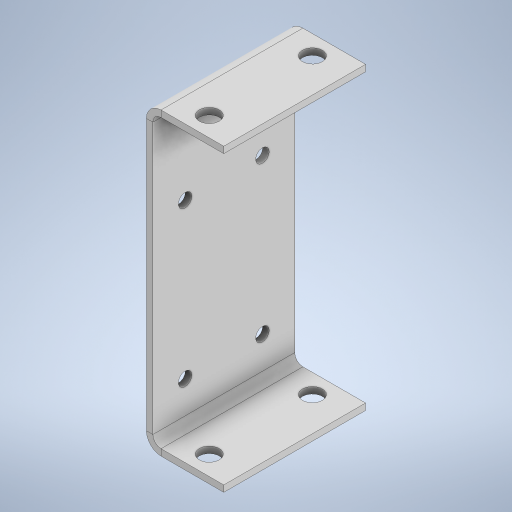
# Autodesk Inventor part: MotorSoport
Saved by Autodesk Inventor 2023.1 (Build 271208000, 208)
## iProperties
Created: 2022-09-08
Part Number: MotorSoport
Material: Genérico
Document SubType Name: Sheet Metal
Designer: Lab. de Manufactura
Density: 1 g/cm^3
Sheet Metal Rule: Por defecto_mm
Appearance: Valor por defecto
Flat Pattern Width: 2.2 cm
Flat Pattern Length: 6.67921 cm
Flat Pattern Area: 14.6943 cm^2
Sheet Metal Width: 22,000 mm
Sheet Metal Length: 66,792 mm
Sheet Metal Area: 1469,427 mm^2
Author: Lab. de Manufactura
Autodesk Inventor part; units mm, degrees
ref_plane "YZ Plane" through (0, 0, 0) normal (1, 0, 0) x (0, 1, 0)
ref_plane "XZ Plane" through (0, 0, 0) normal (0, 1, 0) x (-1, 0, 0)
ref_plane "XY Plane" through (0, 0, 0) normal (0, 0, 1) x (1, 0, 0)
sketch "Boceto1" plane through (0, 0, 0) normal (1, 0, 0) x (0, 1, 0)
  line L0 (0, 0) -> (46.5, 0)
  line L1 (46.5, 0) -> (46.5, -22)
  line L2 (46.5, -22) -> (0, -22)
  line L3 (0, -22) -> (0, 0)
  dimension "d0" = 46.5
  dimension "d1" = 22
  measures "d0" distance of L1.end L2.end
  measures "d1" distance of L0.end L1.end
extrude "Placa1" add sketch "Boceto1" along normal blind 1
sketch "Boceto2" plane through (0, 45.5, 0) normal (0, 1, 0) x (-1, 0, 0)
  line L0 (0, -22) -> (0, 0)
  line L1 (0, 0) -> (-12, 0)
  line L2 (-12, 0) -> (-12, -22)
  line L3 (-12, -22) -> (0, -22)
  constraints: 6 end point, 1 horizontal, 1 perpendicular, 1 vertical
edge flange "Pestaña1" height 12 angle 90 thickness 1 bend radius 1.27 thickness toward (0, 1, 0) relief tear relief width 1 relief depth 0.5 corner gap 1 corner form 0 edges at (1, 46.5, -11) (1, 0, -11) wall of the first edge with corners at (0, 45.5, -22) (0, 45.5, 0) (12, 45.5, 0) (12, 45.5, -22)
bend "Doblez1"
corner "Esquina1"
sketch "Boceto3" plane through (1, 0, 0) normal (1, 0, 0) x (0, 0, -1)
  circle A0 centre (17, 7.25) radius 1.05
  line L0 (0, 0) -> (22, 0) projected
  line L1 (0, 2.27) -> (0, 44.23) projected
  line L2 (0, 0) -> (22, 0) construction
  line L3 (11, 0) -> (11, 46.5) construction
  line L4 (22, 46.5) -> (0, 46.5) construction
  circle A1 centre (5, 7.25) radius 1.05
  line L5 (22, 44.23) -> (22, 2.27) projected
  circle A2 centre (17, 31.25) radius 1.05
  circle A3 centre (5, 31.25) radius 1.05
  dimension "d13" = 2.1
  dimension "d14" = 7.25
  dimension "d16" = 2.1
  dimension "d20" = 24
  dimension "d27" = 12
  dimension "d28" = 6
  constraints: 4 centre point, 2 end point, 2 midpoint, 1 horizontal alignment, 1 vertical, 4 other
  measures "d13" diameter of A0
  measures "d14" distance from line of L0 A0.centre
  measures "d16" diameter of A1
  measures "d20" distance of A0.centre A2.centre
  measures "d27" distance of A0.centre A1.centre
  measures "d28" distance from line of L3 A1.centre
extrude "Cortar1" cut sketch "Boceto3" against normal blind 1
sketch "Boceto4" plane through (12, 1, 0) normal (0, 1, 0) x (1, 0, 0)
  circle A0 centre (-5.25, 19) radius 1.55
  line L0 (-9.73, 22) -> (0, 22) projected
  line L1 (0, 0) -> (0, 22) construction
  line L2 (0, 11) -> (-13.2221, 11) construction
  circle A1 centre (-5.25, 3) radius 1.55
  point P0 (-12, 0)
  point P1 (-12, 22)
  dimension "d29" = 3.1
  dimension "d32" = 3
  dimension "d33" = 6.75
  constraints: 2 centre point, 2 end point, 1 horizontal, 1 midpoint, 1 symmetric about line, 1 other
  measures "d29" diameter of A0
  measures "d32" distance from line of L0 A0.centre
  measures "d33" horizontal distance of point (-12, 22) A0.centre
extrude "Extrusión1" cut sketch "Boceto4" along normal through all both and the other way through all
equation "\"d25\" = Grosor"
equation "\"d2\" = Grosor"
equation "\"d3\" = Anchura_desahogo_plegado"
equation "\"d4\" = Profundidad_desahogo_plegado"
equation "\"d5\" = Remanente_mínimo"
equation "\"d6\" = Radiodetransición"
equation "\"d10\" = Tamaño_destalonado"
equation "\"d11\" = TamañoSeparación"
equation "\"d12\" = Tamaño_de_radio_de_Jacobi"
equation "\"Radio_pliegue\" = Grosor"
equation "\"Anchura_desahogo_plegado\" = Grosor"
equation "\"Profundidad_desahogo_plegado\" = 0.5 * Grosor"
equation "\"Tamaño_destalonado\" = 4 * Grosor"
equation "\"Remanente_mínimo\" = 2 * Grosor"
equation "\"Radiodetransición\" = Radio_pliegue"
equation "\"Tamaño_de_radio_de_Jacobi\" = Radio_pliegue"
equation "\"TamañoSeparación\" = Grosor"
equation "\"Grosor\" = 1"
